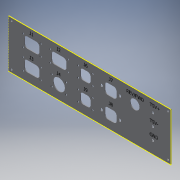
# Autodesk Inventor part: LFEV2017_TSI_006
Saved by Autodesk Inventor 2017 (Build 210142000, 142)
## iProperties
Created: 2017-03-08
Part Number: LFEV2017_TSI_006
Material: Generic
Document SubType Name: Modeling
Designer: hoeflinc
Density: 1 g/cm^3
Appearance: Default
Quantity: 1
Author: hoeflinc
Autodesk Inventor part; units mm, degrees
ref_plane "YZ Plane" through (0, 0, 0) normal (1, 0, 0) x (0, 1, 0)
ref_plane "XZ Plane" through (0, 0, 0) normal (0, 1, 0) x (-1, 0, 0)
ref_plane "XY Plane" through (0, 0, 0) normal (0, 0, 1) x (1, 0, 0)
sketch "Sketch1" plane through (0, 0, 0) normal (0, 0, 1) x (1, 0, 0)
  line L0 (0, 0) -> (342.9, 0)
  line L1 (342.9, 0) -> (342.9, 101.6)
  line L2 (342.9, 101.6) -> (0, 101.6)
  line L3 (0, 101.6) -> (0, 0)
  dimension "d0" = 101.6
  dimension "d1" = 342.9
  constraints: 8 end point, 2 parallel, 1 horizontal, 1 perpendicular
  measures "d0" distance of L2.end L0.start
  measures "d1" distance of L0.start L0.end
extrude "Extrusion1" add sketch "Sketch1" along normal blind 1.5875
sketch "Sketch2" plane through (0, 0, 1.5875) normal (0, 0, 1) x (1, 0, 0)
  line L0 (25.4, 55.245) -> (73.2155, 55.245)
  line L1 (73.2155, 55.245) -> (73.2155, 88.9)
  line L2 (73.2155, 88.9) -> (25.4, 88.9)
  line L3 (25.4, 88.9) -> (25.4, 55.245)
  line L4 (39.6748, 60.8584) -> (58.9407, 60.8584)
  line L5 (65.2907, 67.2084) -> (65.2907, 76.9366)
  line L6 (58.9407, 83.2866) -> (39.6748, 83.2866)
  line L7 (33.3248, 76.9366) -> (33.3248, 67.2084)
  line L8 (0, 101.6) -> (0, 0) projected
  line L9 (342.9, 101.6) -> (0, 101.6) projected
  circle A0 centre (30.48, 83.82) radius 2.0828
  circle A1 centre (68.1355, 83.82) radius 2.0828
  circle A2 centre (68.1355, 60.325) radius 2.0828
  circle A3 centre (30.48, 58.7756) radius 2.0828
  arc A4 (39.6748, 83.2866) -> (33.3248, 76.9366) centre (39.6748, 76.9366) ccw
  arc A5 (33.3248, 67.2084) -> (39.6748, 60.8584) centre (39.6748, 67.2084) ccw
  arc A6 (58.9407, 60.8584) -> (65.2907, 67.2084) centre (58.9407, 67.2084) ccw
  arc A7 (65.2907, 76.9366) -> (58.9407, 83.2866) centre (58.9407, 76.9366) ccw
  point P0 (33.3248, 60.8584)
  point P1 (65.2907, 60.8584)
  point P2 (33.3248, 83.2866)
  dimension "d4" = 33.655
  dimension "d5" = 47.8155
  dimension "d6" = 22.4282
  dimension "d7" = 31.9659
  dimension "d8" = 7.9248
  dimension "d9" = 5.6134
  dimension "d10" = 25.4
  dimension "d11" = 12.7
  dimension "d12" = 4.1656
  dimension "d13" = 5.08
  dimension "d14" = 5.08
  dimension "d15" = 5.08
  dimension "d16" = 5.08
  dimension "d17" = 5.08
  dimension "d18" = 5.08
  dimension "d19" = 5.08
  dimension "d20" = 6.35
  constraints: 16 end point, 9 tangent, 8 centre point, 8 point on circle, 6 equal radius, 6 point on line, 4 parallel, 2 horizontal, 2 perpendicular
  measures "d4" distance of L2.end L0.start
  measures "d5" distance of L0.start L0.end
  measures "d6" distance of point (33.325, 83.287) point (33.325, 60.858)
  measures "d7" distance of point (33.325, 60.858) point (65.291, 60.858)
  measures "d8" distance between parallel lines of L3 L7
  measures "d9" distance between parallel lines of L0 L4
  measures "d10" distance between parallel lines of L8 L3
  measures "d11" distance between parallel lines of L2 L9
  measures "d12" diameter of A0
  measures "d13" distance from line of A0.centre L3
  measures "d14" distance from line of A0.centre L2
  measures "d15" distance from line of L2 A1.centre
  measures "d16" distance from line of A1.centre L1
  measures "d17" distance from line of L1 A2.centre
  measures "d18" distance from line of A2.centre L0
  measures "d19" distance from line of L3 A3.centre
  measures "d20" radius of A4
extrude "Extrusion2" cut sketch "Sketch2" against normal through all contours A5 L7 A4 L6 A7 L5 A6 L4 | A0 | A1 | A2 | A3
pattern_linear "Rectangular Pattern2" count 2 spacing 43.18 along (0, -1, 0) of "Extrusion2"
pattern_linear "Rectangular Pattern3" count 2 spacing 57.15 along (1, 0, 0) of "Extrusion2"
sketch "Sketch3" plane through (0, 0, 1.5875) normal (0, 0, 1) x (1, 0, 0)
  line L0 (0, 101.6) -> (0, 0) construction
  line L1 (342.9, 0) -> (342.9, 101.6) construction
  line L2 (342.9, 101.6) -> (0, 101.6) construction
  line L3 (44.45, 95.3581) -> (52.0207, 95.3581) construction
  line L4 (52.0207, 95.3581) -> (52.0207, 88.9) construction
  line L5 (52.0207, 88.9) -> (44.45, 88.9) construction
  line L6 (44.45, 88.9) -> (44.45, 95.3581) construction
  line L7 (101.6, 95.4713) -> (111.4069, 95.4713) construction
  line L8 (111.4069, 95.4713) -> (111.4069, 88.9) construction
  line L9 (111.4069, 88.9) -> (101.6, 88.9) construction
  line L10 (101.6, 88.9) -> (101.6, 95.4713) construction
  line L11 (44.45, 51.0091) -> (52.8287, 51.0091) construction
  line L12 (52.8287, 51.0091) -> (52.8287, 44.3915) construction
  line L13 (52.8287, 44.3915) -> (44.45, 44.3915) construction
  line L14 (44.45, 44.3915) -> (44.45, 51.0091) construction
  line L15 (101.6, 50.829) -> (109.3588, 50.829) construction
  line L16 (109.3588, 50.829) -> (109.3588, 44.3915) construction
  line L17 (109.3588, 44.3915) -> (101.6, 44.3915) construction
  line L18 (101.6, 44.3915) -> (101.6, 50.829) construction
  line L19 (158.75, 95.5021) -> (171.9813, 95.5021) construction
  line L20 (171.9813, 95.5021) -> (171.9813, 88.9) construction
  line L21 (171.9813, 88.9) -> (158.75, 88.9) construction
  line L22 (158.75, 88.9) -> (158.75, 95.5021) construction
  line L23 (158.75, 50.9937) -> (175.5906, 50.9937) construction
  line L24 (175.5906, 50.9937) -> (175.5906, 44.3915) construction
  line L25 (175.5906, 44.3915) -> (158.75, 44.3915) construction
  line L26 (158.75, 44.3915) -> (158.75, 50.9937) construction
  line L27 (212.09, 95.3375) -> (223.1557, 95.3375) construction
  line L28 (223.1557, 95.3375) -> (223.1557, 88.9) construction
  line L29 (223.1557, 88.9) -> (212.09, 88.9) construction
  line L30 (212.09, 88.9) -> (212.09, 95.3375) construction
  line L31 (212.09, 51.0297) -> (221.933, 51.0297) construction
  line L32 (221.933, 51.0297) -> (221.933, 44.3915) construction
  line L33 (221.933, 44.3915) -> (212.09, 44.3915) construction
  line L34 (212.09, 44.3915) -> (212.09, 51.0297) construction
  constraints: 16 other
sketch "Sketch4" plane through (0, 0, 1.5875) normal (0, 0, 1) x (1, 0, 0)
  line L0 (86.36, 12.7) -> (126.873, 12.7)
  line L1 (126.873, 12.7) -> (126.873, 44.45)
  line L2 (126.873, 44.45) -> (86.36, 44.45)
  line L3 (86.36, 44.45) -> (86.36, 12.7)
  circle A0 centre (91.4146, 39.8018) radius 2.0828
  circle A1 centre (121.793, 39.8018) radius 2.0828
  circle A2 centre (121.793, 17.3482) radius 2.0828
  circle A3 centre (91.4146, 17.3482) radius 2.0828
  circle A4 centre (106.6038, 28.575) radius 12.7
  circle A5 centre (87.63, 58.7756) radius 2.0828 projected
  circle A6 centre (125.2855, 83.82) radius 2.0828 projected
  circle A7 centre (87.63, 83.82) radius 2.0828 projected
  circle A8 centre (125.2855, 60.325) radius 2.0828 projected
  arc A9 (90.4748, 67.2084) -> (96.8248, 60.8584) centre (96.8248, 67.2084) ccw projected
  line L4 (90.4748, 67.2084) -> (90.4748, 76.9366) projected
  arc A10 (96.8248, 83.2866) -> (90.4748, 76.9366) centre (96.8248, 76.9366) ccw projected
  line L5 (96.8248, 83.2866) -> (116.0907, 83.2866) projected
  arc A11 (122.4407, 76.9366) -> (116.0907, 83.2866) centre (116.0907, 76.9366) ccw projected
  line L6 (122.4407, 76.9366) -> (122.4407, 67.2084) projected
  arc A12 (116.0907, 60.8584) -> (122.4407, 67.2084) centre (116.0907, 67.2084) ccw projected
  line L7 (116.0907, 60.8584) -> (96.8248, 60.8584) projected
  circle A13 centre (30.48, 15.5956) radius 2.0828 projected
  circle A14 centre (68.1355, 40.64) radius 2.0828 projected
  circle A15 centre (30.48, 40.64) radius 2.0828 projected
  circle A16 centre (68.1355, 17.145) radius 2.0828 projected
  arc A17 (33.3248, 24.0284) -> (39.6748, 17.6784) centre (39.6748, 24.0284) ccw projected
  line L8 (33.3248, 24.0284) -> (33.3248, 33.7566) projected
  arc A18 (39.6748, 40.1066) -> (33.3248, 33.7566) centre (39.6748, 33.7566) ccw projected
  line L9 (39.6748, 40.1066) -> (58.9407, 40.1066) projected
  arc A19 (65.2907, 33.7566) -> (58.9407, 40.1066) centre (58.9407, 33.7566) ccw projected
  line L10 (65.2907, 33.7566) -> (65.2907, 24.0284) projected
  arc A20 (58.9407, 17.6784) -> (65.2907, 24.0284) centre (58.9407, 24.0284) ccw projected
  line L11 (58.9407, 17.6784) -> (39.6748, 17.6784) projected
  circle A21 centre (30.48, 58.7756) radius 2.0828 projected
  circle A22 centre (68.1355, 83.82) radius 2.0828 projected
  circle A23 centre (30.48, 83.82) radius 2.0828 projected
  circle A24 centre (68.1355, 60.325) radius 2.0828 projected
  arc A25 (33.3248, 67.2084) -> (39.6748, 60.8584) centre (39.6748, 67.2084) ccw projected
  line L12 (33.3248, 67.2084) -> (33.3248, 76.9366) projected
  arc A26 (39.6748, 83.2866) -> (33.3248, 76.9366) centre (39.6748, 76.9366) ccw projected
  line L13 (39.6748, 83.2866) -> (58.9407, 83.2866) projected
  arc A27 (65.2907, 76.9366) -> (58.9407, 83.2866) centre (58.9407, 76.9366) ccw projected
  line L14 (65.2907, 76.9366) -> (65.2907, 67.2084) projected
  arc A28 (58.9407, 60.8584) -> (65.2907, 67.2084) centre (58.9407, 67.2084) ccw projected
  line L15 (58.9407, 60.8584) -> (39.6748, 60.8584) projected
  line L16 (0, 0) -> (342.9, 0) projected
  line L17 (342.9, 0) -> (342.9, 101.6) projected
  line L18 (342.9, 101.6) -> (0, 101.6) projected
  line L19 (0, 101.6) -> (0, 0) projected
  dimension "d53" = 40.513
  dimension "d54" = 31.75
  dimension "d55" = 4.1656
  dimension "d56" = 25.4
  dimension "d57" = 15.875
  dimension "d58" = 15.1892
  dimension "d59" = 15.1892
  dimension "d60" = 15.1892
  dimension "d61" = 15.1892
  dimension "d66" = 11.2268
  dimension "d67" = 11.2268
  dimension "d68" = 11.2268
  dimension "d69" = 11.2268
  dimension "d70" = 5.08
  dimension "d72" = 12.7
  dimension "d207" = 86.36
  constraints: 8 end point, 5 centre point, 3 equal radius, 2 parallel, 1 horizontal, 1 perpendicular
  measures "d53" distance between parallel lines of L1 L3
  measures "d54" distance of L0.end L1.end
  measures "d55" diameter of A0
  measures "d56" diameter of A4
  measures "d57" distance from line of L2 A4.centre
  measures "d58" horizontal distance of A4.centre A3.centre
  measures "d59" horizontal distance of A4.centre A2.centre
  measures "d60" horizontal distance of A0.centre A4.centre
  measures "d61" horizontal distance of A1.centre A4.centre
  measures "d66" vertical distance of A4.centre A2.centre
  measures "d67" vertical distance of A4.centre A3.centre
  measures "d68" vertical distance of A4.centre A0.centre
  measures "d69" vertical distance of A4.centre A1.centre
  measures "d70" distance from line of A1.centre L1
  measures "d72" distance between parallel lines of L0 L16
  measures "d207" distance between parallel lines of L19 L3
extrude "Extrusion3" cut sketch "Sketch4" against normal through all contours A0 | A1 | A2 | A3 | A4
sketch "Sketch5" plane through (0, 0, 1.5875) normal (0, 0, 1) x (1, 0, 0)
  line L0 (142.24, 56.388) -> (182.753, 56.388)
  line L1 (182.753, 56.388) -> (182.753, 88.138)
  line L2 (182.753, 88.138) -> (142.24, 88.138)
  line L3 (142.24, 88.138) -> (142.24, 56.388)
  line L4 (0, 101.6) -> (0, 0) projected
  line L5 (342.9, 101.6) -> (0, 101.6) projected
  circle A0 centre (147.32, 83.4898) radius 2.0828
  circle A1 centre (177.673, 83.4898) radius 2.0828
  circle A2 centre (177.673, 61.0362) radius 2.0828
  circle A3 centre (147.32, 61.0362) radius 2.0828
  line L6 (157.8102, 61.7728) -> (167.2082, 61.7728)
  line L7 (173.5582, 68.1228) -> (173.5582, 76.4032)
  line L8 (167.2082, 82.7532) -> (157.8102, 82.7532)
  line L9 (151.4602, 76.4032) -> (151.4602, 68.1228)
  arc A4 (157.8102, 82.7532) -> (151.4602, 76.4032) centre (157.8102, 76.4032) ccw
  arc A5 (151.4602, 68.1228) -> (157.8102, 61.7728) centre (157.8102, 68.1228) ccw
  arc A6 (167.2082, 61.7728) -> (173.5582, 68.1228) centre (167.2082, 68.1228) ccw
  arc A7 (173.5582, 76.4032) -> (167.2082, 82.7532) centre (167.2082, 76.4032) ccw
  point P0 (151.4602, 61.7728)
  point P1 (173.5582, 82.7532)
  point P2 (151.4602, 82.7532)
  dimension "d95" = 40.513
  dimension "d96" = 31.75
  dimension "d97" = 142.24
  dimension "d98" = 13.462
  dimension "d99" = 4.1656
  dimension "d100" = 5.08
  dimension "d101" = 5.08
  dimension "d102" = 5.08
  dimension "d103" = 5.08
  dimension "d104" = 22.098
  dimension "d105" = 20.9804
  dimension "d106" = 4.1402
  dimension "d107" = 0.7366
  dimension "d108" = 4.6482
  dimension "d109" = 4.6482
  dimension "d110" = 4.6482
  dimension "d111" = 4.6482
  dimension "d112" = 6.35
  dimension "d113" = 4.1148
  constraints: 16 end point, 8 centre point, 8 point on circle, 8 tangent, 6 equal radius, 6 point on line, 4 parallel, 2 horizontal, 2 perpendicular
  measures "d95" distance between parallel lines of L1 L3
  measures "d96" distance of L0.end L1.end
  measures "d97" distance between parallel lines of L4 L3
  measures "d98" distance between parallel lines of L5 L2
  measures "d99" diameter of A0
  measures "d100" distance from line of L3 A0.centre
  measures "d101" distance from line of L3 A3.centre
  measures "d102" distance from line of L1 A2.centre
  measures "d103" distance from line of L1 A1.centre
  measures "d104" distance of point (173.558, 82.753) point (151.46, 82.753)
  measures "d105" distance of point (151.46, 82.753) point (151.46, 61.773)
  measures "d106" distance from line of A0.centre L9
  measures "d107" distance from line of A0.centre L8
  measures "d108" distance from line of A0.centre L2
  measures "d109" distance from line of L0 A3.centre
  measures "d110" distance from line of A2.centre L0
  measures "d111" distance from line of L2 A1.centre
  measures "d112" radius of A4
  measures "d113" distance from line of A1.centre L7
extrude "Extrusion4" cut sketch "Sketch5" against normal through all contours A0 | A1 | A2 | A3 | A5 L9 A4 L8 A7 L7 A6 L6
pattern_linear "Rectangular Pattern4" count 2 spacing 43.942 along (0, -1, 0) of "Extrusion4"
sketch "Sketch6" plane through (0, 0, 1.5875) normal (0, 0, 1) x (1, 0, 0)
  line L0 (209.4738, 61.087) -> (222.1992, 61.087)
  line L1 (228.5492, 67.437) -> (228.5492, 76.835)
  line L2 (222.1992, 83.185) -> (209.4738, 83.185)
  line L3 (203.1238, 76.835) -> (203.1238, 67.437)
  arc A0 (203.1238, 67.437) -> (209.4738, 61.087) centre (209.4738, 67.437) ccw
  arc A1 (222.1992, 61.087) -> (228.5492, 67.437) centre (222.1992, 67.437) ccw
  arc A2 (228.5492, 76.835) -> (222.1992, 83.185) centre (222.1992, 76.835) ccw
  arc A3 (209.4738, 83.185) -> (203.1238, 76.835) centre (209.4738, 76.835) ccw
  circle A4 centre (196.5325, 72.136) radius 2.8067
  circle A5 centre (235.1405, 72.136) radius 2.8067
  line L4 (187.96, 56.642) -> (242.697, 56.642)
  line L5 (242.697, 56.642) -> (242.697, 87.63)
  line L6 (242.697, 87.63) -> (187.96, 87.63)
  line L7 (187.96, 87.63) -> (187.96, 56.642)
  line L8 (342.9, 101.6) -> (0, 101.6) projected
  line L9 (0, 101.6) -> (0, 0) projected
  dimension "d121" = 6.35
  dimension "d122" = 25.4254
  dimension "d123" = 22.098
  dimension "d124" = 5.6134
  dimension "d125" = 5.6134
  dimension "d126" = 6.5913
  dimension "d127" = 6.5913
  dimension "d128" = 11.049
  dimension "d129" = 11.049
  dimension "d130" = 54.737
  dimension "d131" = 30.988
  dimension "d132" = 15.494
  dimension "d133" = 14.1478
  dimension "d134" = 13.97
  dimension "d135" = 187.96
  constraints: 16 end point, 8 point on circle, 8 tangent, 6 centre point, 4 parallel, 3 equal radius, 2 horizontal, 2 perpendicular
  measures "d121" radius of A0
  measures "d122" distance between parallel lines of L1 L3
  measures "d123" distance between parallel lines of L2 L0
  measures "d124" diameter of A4
  measures "d125" diameter of A5
  measures "d126" distance from line of A4.centre L3
  measures "d127" distance from line of A5.centre L1
  measures "d128" distance from line of A4.centre L2
  measures "d129" distance from line of L2 A5.centre
  measures "d130" distance of L6.end L5.end
  measures "d131" distance of L5.end L5.start
  measures "d132" distance from line of A4.centre L6
  measures "d133" distance between parallel lines of L1 L5
  measures "d134" distance between parallel lines of L8 L6
  measures "d135" distance between parallel lines of L9 L7
extrude "Extrusion5" cut sketch "Sketch6" against normal through all contours A0 L3 A3 L2 A2 L1 A1 L0 | A4 | A5
pattern_linear "Rectangular Pattern5" count 2 spacing 44.45 along (0, -1, 0) of "Extrusion5"
sketch "Sketch7" plane through (0, 0, 1.5875) normal (0, 0, 1) x (1, 0, 0)
  circle A0 centre (304.8, 50.8) radius 2.5
  circle A1 centre (304.8, 76.2) radius 2.5
  circle A2 centre (304.8, 25.4) radius 2.5
  line L0 (342.9, 0) -> (342.9, 101.6) projected
  line L1 (342.9, 101.6) -> (0, 101.6) projected
  point P0 (0, 0)
  dimension "d143" = 5
  dimension "d144" = 38.1
  dimension "d145" = 38.1
  dimension "d146" = 38.1
  dimension "d147" = 50.8
  dimension "d148" = 25.4
  dimension "d149" = 76.2
  constraints: 3 centre point, 2 equal radius
  measures "d143" diameter of A0
  measures "d144" distance from line of L0 A0.centre
  measures "d145" distance from line of L0 A1.centre
  measures "d146" distance from line of L0 A2.centre
  measures "d147" distance from line of L1 A0.centre
  measures "d148" distance from line of L1 A1.centre
  measures "d149" distance from line of L1 A2.centre
extrude "Extrusion6" cut sketch "Sketch7" against normal through all
sketch "Sketch8" plane through (0, 0, 1.5875) normal (0, 0, 1) x (1, 0, 0)
  circle A0 centre (266.7, 72.39) radius 10.16
  line L0 (0, 0) -> (342.9, 0) projected
  line L1 (342.9, 101.6) -> (0, 101.6) projected
  line L2 (342.9, 0) -> (342.9, 101.6) projected
  dimension "d152" = 20.32
  dimension "d153" = 101.6
  dimension "d154" = 29.21
  dimension "d155" = 76.2
  constraints: 1 centre point
  measures "d152" diameter of A0
  measures "d153" distance between parallel lines of L0 L1
  measures "d154" distance from line of A0.centre L1
  measures "d155" distance from line of A0.centre L2
extrude "Extrusion7" cut sketch "Sketch8" against normal through all
sketch "Sketch9" plane through (0, 0, 1.5875) normal (0, 0, 1) x (1, 0, 0)
  line L0 (248.92, 92.7572) -> (288.1264, 92.7572) construction
  line L1 (288.1264, 92.7572) -> (288.1264, 82.2059) construction
  line L2 (288.1264, 82.2059) -> (248.92, 82.2059) construction
  line L3 (248.92, 82.2059) -> (248.92, 92.7572) construction
  line L4 (298.45, 92.7572) -> (320.5737, 92.7572) construction
  line L5 (320.5737, 92.7572) -> (320.5737, 83.6558) construction
  line L6 (320.5737, 83.6558) -> (298.45, 83.6558) construction
  line L7 (298.45, 83.6558) -> (298.45, 92.7572) construction
  line L8 (298.45, 63.5) -> (318.5753, 63.5) construction
  line L9 (318.5753, 63.5) -> (318.5753, 55.7178) construction
  line L10 (318.5753, 55.7178) -> (298.45, 55.7178) construction
  line L11 (298.45, 55.7178) -> (298.45, 63.5) construction
  line L12 (298.45, 38.1) -> (316.0334, 38.1) construction
  line L13 (316.0334, 38.1) -> (316.0334, 29.1139) construction
  line L14 (316.0334, 29.1139) -> (298.45, 29.1139) construction
  line L15 (298.45, 29.1139) -> (298.45, 38.1) construction
  line L16 (342.9, 0) -> (342.9, 101.6) projected
  line L17 (342.9, 101.6) -> (0, 101.6) projected
  line L18 (0, 0) -> (342.9, 0) projected
  constraints: 8 other
sketch "Sketch10" plane through (0, 0, 1.5875) normal (0, 0, 1) x (1, 0, 0)
  circle A0 centre (6.35, 95.25) radius 2.0828
  circle A1 centre (6.35, 6.35) radius 2.0828
  circle A2 centre (336.55, 6.35) radius 2.0828
  circle A3 centre (336.55, 95.25) radius 2.0828
  line L0 (342.9, 0) -> (342.9, 101.6) projected
  line L1 (342.9, 101.6) -> (0, 101.6) projected
  line L2 (0, 0) -> (342.9, 0) projected
  line L3 (0, 101.6) -> (0, 0) projected
  dimension "d179" = 4.1656
  dimension "d180" = 6.35
  dimension "d181" = 6.35
  dimension "d182" = 6.35
  dimension "d183" = 6.35
  dimension "d184" = 6.35
  dimension "d185" = 6.35
  dimension "d186" = 6.35
  dimension "d187" = 6.35
  constraints: 4 centre point, 3 equal radius
  measures "d179" diameter of A0
  measures "d180" distance from line of L0 A3.centre
  measures "d181" distance from line of L1 A3.centre
  measures "d182" distance from line of L0 A2.centre
  measures "d183" distance from line of A2.centre L2
  measures "d184" distance from line of A1.centre L2
  measures "d185" distance from line of A1.centre L3
  measures "d186" distance from line of L1 A0.centre
  measures "d187" distance from line of L3 A0.centre
extrude "Extrusion8" cut sketch "Sketch10" against normal through all contours A0 | A1 | A2 | A3
thread "Thread1" size "8-32 UNC" class "2B" standard "ANSI Unified Screw Threads" full length
thread "Thread2" size "8-32 UNC" class "2B" standard "ANSI Unified Screw Threads" full length
thread "Thread3" size "8-32 UNC" class "2B" standard "ANSI Unified Screw Threads" full length
thread "Thread4" size "8-32 UNC" class "2B" standard "ANSI Unified Screw Threads" full length
thread "Thread5" size "8-32 UNC" class "2B" standard "ANSI Unified Screw Threads" full length
thread "Thread6" size "8-32 UNC" class "2B" standard "ANSI Unified Screw Threads" full length
thread "Thread7" size "8-32 UNC" class "2B" standard "ANSI Unified Screw Threads" full length
thread "Thread8" size "8-32 UNC" class "2B" standard "ANSI Unified Screw Threads" full length
thread "Thread9" size "8-32 UNC" class "2B" standard "ANSI Unified Screw Threads" full length
thread "Thread10" size "8-32 UNC" class "2B" standard "ANSI Unified Screw Threads" full length
thread "Thread11" size "8-32 UNC" class "2B" standard "ANSI Unified Screw Threads" full length
thread "Thread12" size "8-32 UNC" class "2B" standard "ANSI Unified Screw Threads" full length
thread "Thread13" size "8-32 UNC" class "2B" standard "ANSI Unified Screw Threads" full length
thread "Thread14" size "8-32 UNC" class "2B" standard "ANSI Unified Screw Threads" full length
thread "Thread15" size "8-32 UNC" class "2B" standard "ANSI Unified Screw Threads" full length
thread "Thread16" size "8-32 UNC" class "2B" standard "ANSI Unified Screw Threads" full length
thread "Thread17" size "8-32 UNC" class "2B" standard "ANSI Unified Screw Threads" full length
thread "Thread18" size "8-32 UNC" class "2B" standard "ANSI Unified Screw Threads" full length
thread "Thread19" size "8-32 UNC" class "2B" standard "ANSI Unified Screw Threads" full length
thread "Thread20" size "8-32 UNC" class "2B" standard "ANSI Unified Screw Threads" full length
thread "Thread21" size "8-32 UNC" class "2B" standard "ANSI Unified Screw Threads" full length
thread "Thread22" size "8-32 UNC" class "2B" standard "ANSI Unified Screw Threads" full length
thread "Thread23" size "8-32 UNC" class "2B" standard "ANSI Unified Screw Threads" full length
thread "Thread24" size "8-32 UNC" class "2B" standard "ANSI Unified Screw Threads" full length
sketch "Sketch11" plane through (0, 0, 0) normal (0, 0, -1) x (-1, 0, 0)
  line L0 (-285.4519, 43.4444) -> (-249.3971, 43.4444) construction
  line L1 (-249.3971, 43.4444) -> (-249.3971, 39.7196) construction
  line L2 (-249.3971, 39.7196) -> (-285.4519, 39.7196) construction
  line L3 (-285.4519, 39.7196) -> (-285.4519, 43.4444) construction
  point P0 (0, 0)
  constraints: 2 other
equation "\"d8\" = -0.5 * d7 + 0.5 * d5"
equation "\"d9\" = -0.5 * d6 + 0.5 * d4"
equation "\"d15\" = d14"
equation "\"d16\" = d13"
equation "\"d17\" = d16"
equation "\"d18\" = d15"
equation "\"d19\" = d13"
equation "\"d57\" = 0.5 * d54"
equation "\"d59\" = d58"
equation "\"d60\" = d58"
equation "\"d61\" = d60"
equation "\"d67\" = d66"
equation "\"d68\" = d66"
equation "\"d69\" = d66"
equation "\"d101\" = d100"
equation "\"d102\" = d101"
equation "\"d103\" = d100"
equation "\"d109\" = d108"
equation "\"d110\" = d109"
equation "\"d111\" = d108"
equation "\"d128\" = 0.5 * d123"
equation "\"d132\" = 0.5 * d131"
equation "\"d145\" = d144"
equation "\"d146\" = d144"
body "Solid1"
